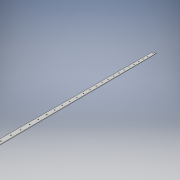
# Autodesk Inventor part: Profile-Flat-01
Saved by Autodesk Inventor 2018 (Build 220112000, 112)
## iProperties
Created: 2025-02-17
Part Number: Profile-Flat-01
Material: Všeobecné
Document SubType Name: Modeling
Designer: Jozko Mrkvicka
Density: 1 g/cm^3
Appearance: Výchozí
Author: Jozko Mrkvicka
Autodesk Inventor part; units mm, degrees
ref_plane "YZ Plane" through (0, 0, 0) normal (1, 0, 0) x (0, 1, 0)
ref_plane "XZ Plane" through (0, 0, 0) normal (0, 1, 0) x (-1, 0, 0)
ref_plane "XY Plane" through (0, 0, 0) normal (0, 0, 1) x (1, 0, 0)
sketch "Náčrt1" plane through (0, 0, 0) normal (0, 0, 1) x (1, 0, 0)
  line L0 (-7.5, -1) -> (7.5, -1)
  line L1 (7.5, -1) -> (7.5, 1)
  line L2 (7.5, 1) -> (-7.5, 1)
  line L3 (-7.5, 1) -> (-7.5, -1)
  line L4 (-7.5, -1) -> (7.5, 1) construction
  line L5 (7.5, -1) -> (-7.5, 1) construction
  point P0 (0, 0)
  dimension "d0" = 15
  dimension "d1" = 2
  constraints: 12 end point, 2 midpoint, 2 parallel, 1 horizontal, 1 perpendicular
  measures "d0" distance of L1.end L2.end
  measures "d1" distance of L0.end L1.end
extrude "Vysunutí1" add sketch "Náčrt1" along normal blind 640
sketch "Náčrt2" plane through (-7.5, 1, 0) normal (0, 1, 0) x (1, 0, 0)
  line L0 (15, 0) -> (0, 0) projected
  line L1 (0, 0) -> (0, -640) projected
  line L2 (15, -640) -> (0, -640) projected
  line L3 (15, 0) -> (15, -640) projected
  circle A0 centre (7.5, -7.5) radius 1.5
  line L4 (15, 0) -> (15, -640) projected
  line L5 (15, -320) -> (0, -320)
  circle A1 centre (7.5, -632.5) radius 1.5
  point P0 (7.5, 0)
  dimension "d4" = 7.5
  dimension "d6" = 7.5
  dimension "d7" = 3
  constraints: 2 centre point, 2 end point, 2 midpoint, 1 symmetric about line, 1 other
  measures "d4" distance from line of A0.centre L0
  measures "d6" horizontal distance of L0.start A0.centre
  measures "d7" diameter of A0
extrude "Vysunutí2" cut sketch "Náčrt2" against normal up to next contours A0 | A1
sketch "Náčrt3" plane through (-7.5, 1, 0) normal (0, 1, 0) x (1, 0, 0)
  line L0 (15, 0) -> (15, -640) projected
  line L1 (0, 0) -> (0, -640) projected
  circle A0 centre (7.5, -320) radius 1.5
  line L2 (15, 0) -> (0, 0) projected
  point P0 (7.5, 0)
  dimension "d11" = 3
  dimension "d12" = 7.5
  dimension "d13" = 320
  constraints: 1 centre point
  measures "d11" diameter of A0
  measures "d12" distance from line of L1 A0.centre
  measures "d13" distance from line of L2 A0.centre
extrude "Vysunutí3" cut sketch "Náčrt3" against normal up to next
pattern_linear "Obdélníkové pole1" count 12 spacing 25.4 along (0, 0, 1) count 12 spacing 25.4 along (0, 0, -1) of "Vysunutí3"
equation "\"d0\" = width"
equation "\"d1\" = thickness"
equation "\"d2\" = length"
equation "\"d4\" = 0.5 * width"
equation "\"d6\" = 0.5 * width"
equation "\"d7\" = holeDia"
equation "\"d8\" = length"
equation "\"d12\" = 0.5 * width"
equation "\"d13\" = 0.5 * length"
equation "\"d14\" = length"
equation "\"d16\" = 0.5 * holeCount"
equation "\"d18\" = holeDistance"
equation "\"d19\" = 0.5 * holeCount"
equation "\"d21\" = holeDistance"
equation "\"length\" = gCabinet_FerriteCore_Width"
equation "\"width\" = 15"
equation "\"thickness\" = 2"
equation "\"holeDia\" = 3"
equation "\"holeDistance\" = 25.4"
equation "\"holeCount\" = 23"
equation "\"gCabinet_FerriteCore_Width\" = 640"
